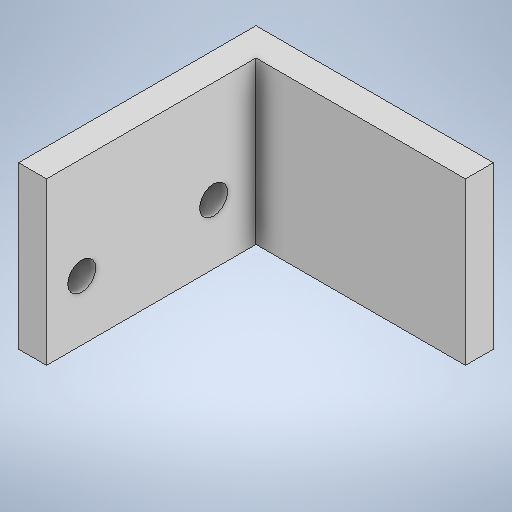
# Autodesk Inventor part: MuteMount
Saved by Autodesk Inventor 2025.1 (Build 291241000, 241)
## iProperties
Created: 2025-12-01
Part Number: MuteMount
Material: Generic
Document SubType Name: Modeling
Designer: Juxin
Density: 1 g/cm^3
Appearance: Default
Author: Juxin
Autodesk Inventor part; units mm, degrees
ref_plane "YZ Plane" through (0, 0, 0) normal (1, 0, 0) x (0, 1, 0)
ref_plane "XZ Plane" through (0, 0, 0) normal (0, 1, 0) x (-1, 0, 0)
ref_plane "XY Plane" through (0, 0, 0) normal (0, 0, 1) x (1, 0, 0)
sketch "Sketch1" plane through (0, 0, 0) normal (0, 1, 0) x (-1, 0, 0)
  line L0 (0, 0) -> (26.9875, 0)
  line L1 (26.9875, 0) -> (26.9875, -26.9875)
  line L2 (26.9875, -26.9875) -> (0, -26.9875)
  line L3 (0, -26.9875) -> (0, 0)
  line L4 (26.9875, -23.3392) -> (23.8125, -23.3392)
  line L5 (0, -23.8125) -> (0, 0)
  line L6 (0, 0) -> (51.181, 0)
  line L7 (23.8125, -26.9875) -> (23.8125, -23.8125)
  line L8 (23.8125, -23.8125) -> (0, -23.8125)
  line L9 (0, -23.8125) -> (0, 0)
  line L10 (0, 0) -> (23.8125, 0)
  line L11 (23.8125, 0) -> (23.8125, -23.8125)
  dimension "d0" = 26.9875
  dimension "d1" = 26.9875
  dimension "d2" = 3.175
  dimension "d4" = 3.175
  constraints: 24 end point, 4 parallel, 3 horizontal, 2 perpendicular, 2 point on line, 1 vertical
  measures "d0" distance of L1.end L2.end
  measures "d1" distance of L0.end L1.end
  measures "d2" distance of L4.start L4.end
  measures "d4" distance of L7.start L7.end
extrude "Extrusion1" add sketch "Sketch1" along normal blind 18.3642 contours L0 L1 L4 L11 | L8 L7 L2 L3 | L4 L1 L2 L7 L11
sketch "Sketch4" plane through (-26.9875, 0, -26.9875) normal (-1, 0, 0) x (0, 0, 1)
  line L0 (26.9875, 0) -> (26.9875, 18.3642) projected
  line L1 (0, 0) -> (26.9875, 0)
  line L2 (26.9875, 0) -> (26.9875, 13.589)
  line L3 (26.9875, 13.589) -> (0, 13.589)
  line L4 (0, 13.589) -> (0, 0)
  line L5 (0, 0) -> (0, 18.3642) projected
  line L6 (0, 6.7945) -> (8.001, 6.7945)
  circle A0 centre (8.001, 6.7945) radius 1.5875
  line L7 (8.001, 6.7945) -> (22.987, 6.7945)
  circle A1 centre (22.987, 6.7945) radius 1.5875
  dimension "d23" = 13.589
  dimension "d24" = 8.001
  dimension "d25" = 3.175
  dimension "d26" = 14.986
  dimension "d27" = 3.175
  constraints: 12 end point, 2 centre point, 2 coincident, 2 horizontal, 2 parallel, 2 perpendicular, 2 point on line
  measures "d23" distance of L2.end L1.end
  measures "d24" distance of L6.start L6.end
  measures "d25" diameter of A0
  measures "d26" distance of L7.start L7.end
  measures "d27" diameter of A1
extrude "Extrusion4" cut sketch "Sketch4" against normal blind 18.3642 contours A0 L7 L6 | L6 L7 A0 | A1
body "Solid1"
